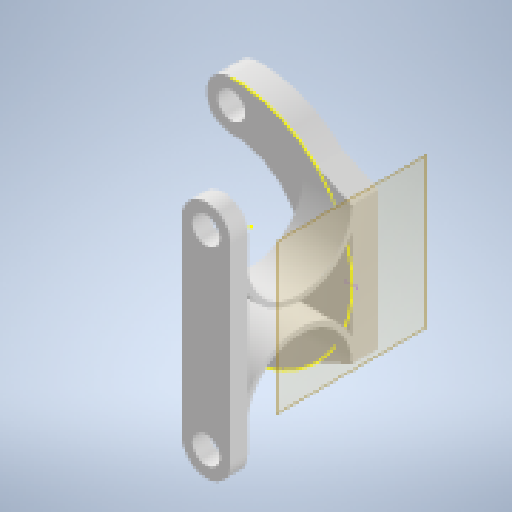
# Autodesk Inventor part: MotorMountTopSuspension
Saved by Autodesk Inventor 2024 (Build 280153020, 153B)
## iProperties
Created: 2024-04-18
Part Number: MotorMountTopSuspension
Material: Generic
Document SubType Name: Modeling
Designer: lvrectanus0
Density: 1 g/cm^3
Appearance: Default
Author: lvrectanus0
Autodesk Inventor part; units mm, degrees
ref_plane "YZ Plane" through (0, 0, 0) normal (1, 0, 0) x (0, 1, 0)
ref_plane "XZ Plane" through (0, 0, 0) normal (0, 1, 0) x (-1, 0, 0)
ref_plane "XY Plane" through (0, 0, 0) normal (0, 0, 1) x (1, 0, 0)
sketch "Sketch1" plane through (0, 0, 0) normal (0, 0, 1) x (1, 0, 0)
  circle A0 centre (-2.8902, -14) radius 2 projected
  line L0 (-2.8902, -17.5998) -> (-2.8902, -19) projected
  line L1 (7.1098, -19) -> (-2.8902, -19) projected
  line L2 (7.1098, -14) -> (7.1098, -19) projected
  line L3 (7.1098, -14) -> (0.6714, -14) projected
  arc A1 (0.6714, -14) -> (-2.8902, -10.4002) centre (-2.9286, -14) ccw projected
  arc A2 (-2.8902, -10.4002) -> (-2.8902, -17.5998) centre (-2.9286, -14) ccw projected
  circle A3 centre (-2.8902, 14) radius 2 projected
  line L4 (-2.8902, 17.5998) -> (-2.8902, 19) projected
  arc A4 (-2.8902, 17.5998) -> (-2.8902, 10.4002) centre (-2.9286, 14) ccw projected
  arc A5 (-2.8902, 10.4002) -> (0.6714, 14) centre (-2.9286, 14) ccw projected
  line L5 (7.1098, 14) -> (0.6714, 14) projected
  line L6 (7.1098, 14) -> (7.1098, 19) projected
  line L7 (7.1098, 19) -> (-2.8902, 19) projected
  line L8 (9.8002, 10) -> (3.5098, 10) projected
  line L9 (-57.6094, 10) -> (18.5906, 10) projected
  arc A6 (-2.8902, -10.4002) -> (-2.8902, 10.4002) centre (-2.7794, 0) ccw
  circle A7 centre (-2.9286, -14) radius 3.6
  circle A8 centre (-2.9286, 14) radius 3.6
  arc A9 (-2.9669, -17.5998) -> (-2.9669, 17.5998) centre (-2.7794, 0) ccw
  point P0 (7.1098, 10)
  point P1 (0, 0)
  point P2 (-2.8902, -17.6004)
  point P3 (-2.8902, 17.6004)
  constraints: 4 point on circle, 2 centre point, 2 coincident, 2 tangent, 1 horizontal alignment, 1 point on line, 9 other
extrude "Extrusion2" add sketch "Sketch1" along normal blind 4 contours A2 A1 A7 | A7 L3 L2 A9 | A1 A6 L9 L8 A9 L2 L3 | L9 L8 A6 A5 L5 L6 A9 | L6 L5 A8 A9 | A4 A8 A5
sketch "Sketch2" plane through (0, 0, 4) normal (0, 0, 1) x (1, 0, 0)
  arc A0 (-2.8902, -17.6004) -> (-2.8902, 17.6004) centre (-2.7794, 0) ccw projected
  point P0 (0, 0)
  point P1 (14.8214, 0)
  constraints: 1 point on circle
ref_plane "Work Plane1" through (14.8214, 0, 4) normal (1, 0, 0) x (0, 1, 0)
sketch "Sketch3" plane through (14.8214, 0, 4) normal (1, 0, 0) x (0, 1, 0)
  line L0 (17.6008, 0) -> (-17.6008, 0) projected
  arc A0 (-10.16, 0) -> (-10.16, 15.24) centre (-10.16, 7.62) ccw
  line L1 (-10.16, 7.62) -> (-10.16, 0) construction
  line L2 (-10.16, 7.62) -> (-2.54, 7.62) construction
  line L3 (-10.16, 7.62) -> (-10.16, 15.24) construction
  arc A1 (-12.6408, -0.4263) -> (-10.96, 16.0019) centre (-10.16, 7.62) ccw
  line L4 (-10.96, 16.0019) -> (-10.96, 9.0533) construction
  line L5 (0, 0) -> (0, 16.929) construction
  line L6 (-10.16, 15.24) -> (0, 15.24)
  line L7 (-10.16, 15.24) -> (-17.6008, 15.24)
  line L8 (-17.6008, 15.24) -> (-17.6008, 17.78)
  line L9 (-17.6008, 17.78) -> (0, 17.78)
  line L10 (-10.16, 0) -> (-10.16, -0.8)
  line L11 (17.6008, -4) -> (-17.6008, -4) projected
  line L12 (-10.16, 0) -> (0, 0)
  line L13 (0, 0) -> (0, -4)
  line L14 (0, -4) -> (-10.16, -4)
  line L15 (-10.16, -4) -> (-10.16, 0)
  arc A2 (10.16, 15.24) -> (10.16, 0) centre (10.16, 7.62) ccw
  line L16 (10.16, 7.62) -> (10.16, 0) construction
  line L17 (10.16, 7.62) -> (2.54, 7.62) construction
  line L18 (10.16, 7.62) -> (10.16, 15.24) construction
  arc A3 (10.96, 16.0019) -> (12.6408, -0.4263) centre (10.16, 7.62) ccw
  line L19 (10.96, 16.0019) -> (10.96, 9.0533) construction
  line L20 (10.16, 15.24) -> (0, 15.24)
  line L21 (10.16, 15.24) -> (17.6008, 15.24)
  line L22 (17.6008, 15.24) -> (17.6008, 17.78)
  line L23 (17.6008, 17.78) -> (0, 17.78)
  line L24 (10.16, 0) -> (10.16, -0.8)
  line L25 (10.16, 0) -> (0, 0)
  line L26 (0, -4) -> (10.16, -4)
  line L27 (10.16, -4) -> (10.16, 0)
  point P0 (-17.6004, 0)
  point P1 (17.6004, 0)
  point P2 (-17.6004, -4)
  point P3 (17.6004, -4)
  point P4 (-6.5778, 0)
  point P5 (-6.5778, 15.24)
  point P6 (6.5778, 15.24)
  point P7 (6.5778, 0)
  dimension "d4" = 90
  dimension "d5" = 180
  dimension "d6" = 0.8
  dimension "d7" = 7.62
  dimension "d8" = 10.16
  dimension "d9" = 2.54
  constraints: 52 end point, 11 symmetric about line, 10 point on circle, 6 perpendicular, 4 centre point, 4 point on line, 2 horizontal, 2 parallel, 1 midpoint, 1 vertical, 1 vertical alignment, 3 other
  measures "d4" angle of L1 L2
  measures "d5" angle of L1 L3
  measures "d6" radial gap between concentric circles of A0 A1
  measures "d7" distance of L1.end L1.start
  measures "d8" distance from line of L1.start L5
  measures "d9" distance of L7.end L8.end
extrude "Extrusion3" add sketch "Sketch3" against normal blind 7.2 contours L24 A3 L0 | L0 A3 L20 A2 | A3 L27 L11 L13 L0 | L20 L6 L7 L8 L9 L23 L22 L21 | L13 L11 L15 A1 L0 | A1 L10 L0 | L0 A0 L6 A1
chamfer "Chamfer1" distance 3.175 angle 45 2 edges at (11.5929, -10.16, 2) (11.5929, 10.16, 2)
fillet "Fillet1" radius 3.6 4 edges at (14.8214, -17.6008, 20.51) (14.8214, 17.6008, 20.51) (7.6214, 17.6008, 20.51) (7.6214, -17.6008, 20.51)
sketch "Sketch4" plane through (14.8214, -14.0008, 21.78) normal (0, 0, 1) x (1, 0, 0)
  arc A0 (-7.2, 0) -> (0, 0) centre (-3.6, 0) ccw projected
  line L0 (0, 28.0016) -> (0, 0) projected
  arc A1 (0, 28.0016) -> (-7.2, 28.0016) centre (-3.6, 28.0016) ccw projected
  line L1 (-7.2, 0) -> (-7.2, 28.0016) projected
  circle A2 centre (-3.6, 0) radius 2
  circle A3 centre (-3.6, 28.0016) radius 2
  point P0 (-14.8214, 14.0008)
  dimension "d16" = 4
  dimension "d17" = 4
  constraints: 2 centre point, 2 coincident
  measures "d16" diameter of A2
  measures "d17" diameter of A3
hole "Hole1" at (11.2214, -14.0008, 21.78) at (11.2214, 14.0008, 21.78) direction (0, 0, -1) diameter 4 depth 6
body "Solid2"
